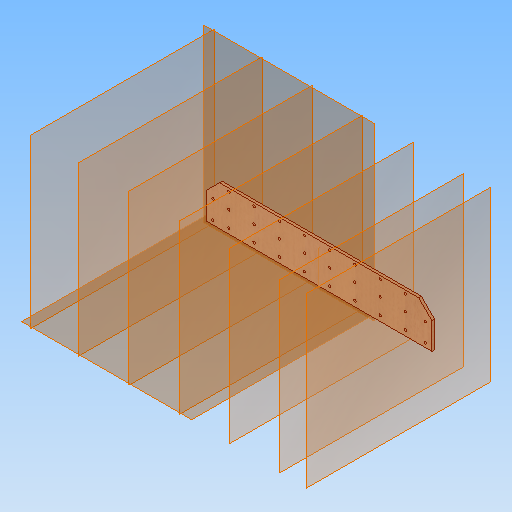
# Autodesk Inventor part: Pancake_Timing Backboard_4 Lanes
Saved by Autodesk Inventor 2018.1 (Build 221171000, 171)
## iProperties
Created: 2019-02-22
Part Number: Pancake_Timing Backboard_4 Lanes
Material: Wood (Oak)
Document SubType Name: Modeling
Designer: James
Density: 0.76 g/cm^3
Appearance: White Oak - Natural Medium Gloss
Mass: 117.058 g
Surface Area: 684.421 cm^2
Volume: 154.023 cm^3
Author: James
Autodesk Inventor part; units mm, degrees
ref_plane "YZ Plane" through (0, 0, 0) normal (1, 0, 0) x (0, 1, 0)
ref_plane "XZ Plane" through (0, 0, 0) normal (0, 1, 0) x (-1, 0, 0)
ref_plane "XY Plane" through (0, 0, 0) normal (0, 0, 1) x (1, 0, 0)
derived "Pancake_Skeleton.ipt"
ref_plane "Ground" through (0, 0, 0) normal (0, 1, 0) x (-1, 0, 0)
ref_plane "Back" through (0, 0, 0) normal (0, 0, 1) x (1, 0, 0)
ref_plane "LHS" through (0, 0, 0) normal (1, 0, 0) x (0, 1, 0)
ref_plane "Lane 1" through (90, 0, 0) normal (1, 0, 0) x (0, 1, 0)
ref_plane "Lane 2" through (185, 0, 0) normal (1, 0, 0) x (0, 1, 0)
ref_plane "Lane 3" through (280, 0, 0) normal (1, 0, 0) x (0, 1, 0)
ref_plane "Lane 4" through (375, 0, 0) normal (1, 0, 0) x (0, 1, 0)
ref_plane "Lane 5" through (470, 0, 0) normal (1, 0, 0) x (0, 1, 0)
ref_plane "RHS" through (520, 0, 0) normal (1, 0, 0) x (0, 1, 0)
sketch "Sketch1" plane through (0, 0, 0) normal (0, 0, 1) x (1, 0, 0)
  line L0 (0, 90) -> (0, -15) projected
  line L1 (-85, 0) -> (510, 0) projected
  line L2 (0, 0) -> (425, 0)
  line L3 (425, 0) -> (425, 75)
  line L4 (425, 75) -> (0, 75)
  line L5 (0, 75) -> (0, 0)
  line L6 (520, 90) -> (520, -15) projected
  dimension "d1" = 75
  dimension "d30" = 95
  constraints: 8 end point, 2 parallel, 1 horizontal, 1 perpendicular
  measures "d1" distance of L2.end L3.end
  measures "d30" distance between parallel lines of L6 L3
extrude "Extrusion1" add sketch "Sketch1" along normal blind 5
sketch "Sketch2" plane through (0, 0, 5) normal (0, 0, 1) x (1, 0, 0)
  line L0 (90, 90) -> (90, -15) projected
  line L1 (425, 75) -> (0, 75) projected
  line L2 (-85, 0) -> (510, 0) projected
  line L3 (185, 90) -> (185, -15) projected
  point P0 (0, 0)
  point P1 (42.5, 40)
  point P2 (42.5, 10)
  point P3 (42.5, 69)
  dimension "d4" = 30
  dimension "d28" = 47.5
  dimension "d29" = 95
  dimension "d31" = 10
  dimension "d32" = 6
  constraints: 2 vertical alignment
  measures "d4" distance of point (42.5, 10) point (42.5, 40)
  measures "d28" distance from line of L0 point (42.5, 40)
  measures "d29" distance between parallel lines of L3 L0
  measures "d31" distance from line of L2 point (42.5, 10)
  measures "d32" distance from line of point (42.5, 69) L1
hole "Hole1" at (42.5, 40, 5) at (42.5, 10, 5) at (42.5, 69, 5) direction (0, 0, -1) diameter 4.5 end through all clearance for "Socket Head Cap Screw" size "M4" standard "Ansi Metric M Profile"
pattern_linear "Rectangular Pattern1" count 8 spacing 47.5 along (1, 0, 0) of "Hole1"
sketch "Sketch3" plane through (0, 0, 5) normal (0, 0, 1) x (1, 0, 0)
  line L0 (425, 75) -> (0, 75) projected
  line L1 (-85, 0) -> (510, 0) projected
  line L2 (0, 90) -> (0, -15) projected
  point P0 (0, 0)
  point P1 (12.5, 42.5)
  point P2 (12.5, 7.5)
  dimension "d17" = 32.5
  dimension "d18" = 7.5
  dimension "d19" = 35
  dimension "d20" = 12.5
  constraints: 1 vertical alignment
  measures "d17" distance from line of L0 point (12.5, 42.5)
  measures "d18" distance from line of L1 point (12.5, 7.5)
  measures "d19" distance of point (12.5, 42.5) point (12.5, 7.5)
  measures "d20" distance from line of L2 point (12.5, 42.5)
hole "Hole2" at (12.5, 42.5, 5) at (12.5, 7.5, 5) direction (0, 0, -1) diameter 4.5 end through all clearance for "Socket Head Cap Screw" size "M4" standard "Ansi Metric M Profile"
ref_plane "Work Plane10" through (212.5, 0, 0) normal (-1, 0, 0) x (0, 0, 1)
mirror "Mirror1" about plane through (212.5, 0, 0) normal (-1, 0, 0) of "Hole2"
chamfer "Chamfer1" distance 25 angle 45 2 edges at (0, 75, 2.5) (425, 75, 2.5)
equation "\"d28\" = 0.5 * d29"
body "Solid1"
